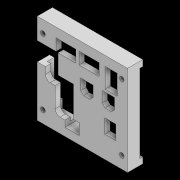
# Autodesk Inventor part: fan_controller_case_top
Saved by Autodesk Inventor 2022 (Build 260153000, 153)
## iProperties
Created: 2022-10-14
Part Number: fan_controller_case_top
Material: 一般
Document SubType Name: Modeling
Designer: numai
Density: 1 g/cm^3
Appearance: 既定
Author: numai
Autodesk Inventor part; units mm, degrees
ref_plane "YZ Plane" through (0, 0, 0) normal (1, 0, 0) x (0, 1, 0)
ref_plane "XZ Plane" through (0, 0, 0) normal (0, 1, 0) x (-1, 0, 0)
ref_plane "XY Plane" through (0, 0, 0) normal (0, 0, 1) x (1, 0, 0)
sketch "スケッチ1" plane through (0, 0, 0) normal (0, 0, 1) x (1, 0, 0)
  line L0 (-25.3, 21.7) -> (25.3, 21.7)
  line L1 (25.3, 21.7) -> (25.3, -21.7)
  line L2 (25.3, -21.7) -> (-25.3, -21.7)
  line L3 (-25.3, -21.7) -> (-25.3, 21.7)
  circle A0 centre (-22.1, 18.5) radius 1.3
  circle A1 centre (22.1, 18.5) radius 1.3
  circle A2 centre (22.1, -18.5) radius 1.3
  circle A3 centre (-22.1, -18.5) radius 1.3
  line L4 (-18.1, 19.2) -> (-18.1, 14.5)
  line L5 (-18.1, 14.5) -> (-22.8, 14.5)
  line L6 (-22.8, 14.5) -> (-22.8, -14.5)
  line L7 (-22.8, -14.5) -> (-18.1, -14.5)
  line L8 (-18.1, -14.5) -> (-18.1, -19.2)
  line L9 (-18.1, -19.2) -> (18.1, -19.2)
  line L10 (18.1, -19.2) -> (18.1, -14.5)
  line L11 (18.1, -14.5) -> (22.8, -14.5)
  line L12 (22.8, -14.5) -> (22.8, 14.5)
  line L13 (22.8, 14.5) -> (18.1, 14.5)
  line L14 (18.1, 14.5) -> (18.1, 19.2)
  line L15 (18.1, 19.2) -> (-18.1, 19.2)
  point P0 (0, 0)
  point P1 (0, 21.7)
  point P2 (-25.3, 0)
  dimension "d0" = 50.6
  dimension "d1" = 43.4
  dimension "d2" = 2.6
  dimension "d3" = 44.2
  dimension "d4" = 37
  dimension "d5" = 22.1
  dimension "d6" = 18.5
  dimension "d7" = 2.5
  dimension "d8" = 2.5
  dimension "d9" = 2.5
  dimension "d10" = 2.5
  dimension "d11" = 4
  dimension "d12" = 4
  dimension "d13" = 4
  dimension "d14" = 4
  dimension "d15" = 4
  constraints: 32 end point, 8 perpendicular, 6 point on line, 4 centre point, 3 equal radius, 3 horizontal alignment, 3 parallel, 3 vertical alignment, 2 midpoint, 1 horizontal, 1 vertical
  measures "d0" distance of L0.start L0.end
  measures "d1" distance of L0.end L1.end
  measures "d2" diameter of A0
  measures "d3" distance of A1.centre A0.centre
  measures "d4" distance of A3.centre A0.centre
  measures "d5" horizontal distance of point (0, 0) A1.centre
  measures "d6" vertical distance of point (0, 0) A0.centre
  measures "d7" distance between parallel lines of L0 L15
  measures "d8" distance between parallel lines of L3 L6
  measures "d9" distance between parallel lines of L2 L9
  measures "d10" distance between parallel lines of L1 L12
  measures "d11" distance from line of L5 A0.centre
  measures "d12" distance from line of L4 A0.centre
  measures "d13" distance from line of L14 A1.centre
  measures "d14" distance from line of A3.centre L7
  measures "d15" distance from line of L10 A2.centre
extrude "押し出し1" add sketch "スケッチ1" along normal blind 6.9
sketch "スケッチ4" plane through (0, 0, 6.9) normal (0, 0, 1) x (1, 0, 0)
  line L0 (-18.1, 14.5) -> (-18.1, 19.2) projected
  line L1 (-18.1, 19.2) -> (18.1, 19.2) projected
  line L2 (-22.8, 14.5) -> (-18.1, 14.5) projected
  line L3 (-22.8, -14.5) -> (-22.8, 14.5) projected
  line L4 (-18.1, -14.5) -> (-22.8, -14.5) projected
  line L5 (-18.1, -19.2) -> (-18.1, -14.5) projected
  line L6 (18.1, -19.2) -> (-18.1, -19.2) projected
  line L7 (18.1, -14.5) -> (18.1, -19.2) projected
  line L8 (22.8, -14.5) -> (18.1, -14.5) projected
  line L9 (22.8, 14.5) -> (22.8, -14.5) projected
  line L10 (18.1, 14.5) -> (22.8, 14.5) projected
  line L11 (18.1, 19.2) -> (18.1, 14.5) projected
  point P0 (0, 0)
extrude "押し出し4" add sketch "スケッチ4" against normal blind 3
sketch "スケッチ3" plane through (0, 0, 6.9) normal (0, 0, 1) x (1, 0, 0)
  line L0 (-14.6, 19.9) -> (-3.9, 19.9) construction
  line L1 (-3.9, 19.9) -> (-3.9, 13.6) construction
  line L2 (-3.9, 13.6) -> (-14.6, 13.6) construction
  line L3 (-14.6, 13.6) -> (-14.6, 19.9) construction
  line L4 (-1.6, 19.9) -> (9.1, 19.9) construction
  line L5 (9.1, 19.9) -> (9.1, 13.6) construction
  line L6 (9.1, 13.6) -> (-1.6, 13.6) construction
  line L7 (-1.6, 13.6) -> (-1.6, 19.9) construction
  line L8 (13, 19.8) -> (19.3, 19.8) construction
  line L9 (19.3, 19.8) -> (19.3, 9.1) construction
  line L10 (19.3, 9.1) -> (13, 9.1) construction
  line L11 (13, 9.1) -> (13, 19.8) construction
  line L12 (25.3, 21.7) -> (-25.3, 21.7) construction
  line L13 (25.3, -21.7) -> (25.3, 21.7) construction
  line L14 (-14.8, 13.4) -> (-3.7, 13.4)
  line L15 (-3.7, 13.4) -> (-3.7, 20.1)
  line L16 (-3.7, 20.1) -> (-14.8, 20.1)
  line L17 (-14.8, 20.1) -> (-14.8, 13.4)
  line L18 (-1.8, 13.4) -> (9.3, 13.4)
  line L19 (9.3, 13.4) -> (9.3, 20.1)
  line L20 (9.3, 20.1) -> (-1.8, 20.1)
  line L21 (-1.8, 20.1) -> (-1.8, 13.4)
  line L22 (12.8, 8.9) -> (19.5, 8.9)
  line L23 (19.5, 8.9) -> (19.5, 20)
  line L24 (19.5, 20) -> (12.8, 20)
  line L25 (12.8, 20) -> (12.8, 8.9)
  point P0 (0, 0)
  dimension "d20" = 6.3
  dimension "d21" = 10.7
  dimension "d23" = 6
  dimension "d24" = 1.8
  dimension "d25" = 26.9
  dimension "d26" = 39.9
  dimension "d27" = 12.6
  dimension "d28" = 0.2
  dimension "d29" = 0.2
  dimension "d30" = 0.2
  constraints: 48 end point, 12 parallel, 6 perpendicular, 3 equal length, 3 horizontal, 2 point on line, 9 other
  measures "d20" distance of L8.start L8.end
  measures "d21" distance of L8.end L9.end
  measures "d23" distance from line of L12.start L9
  measures "d24" distance between parallel lines of L12 L4
  measures "d25" distance between parallel lines of L13 L7
  measures "d26" distance from line of L12.start L3
  measures "d27" distance between parallel lines of L10 L12
  measures "d28" distance between parallel lines of L2 L14
  measures "d29" distance between parallel lines of L6 L18
  measures "d30" distance between parallel lines of L10 L22
extrude "押し出し3" cut sketch "スケッチ3" along normal through all both and the other way through all
sketch "スケッチ5" plane through (0, 0, 6.9) normal (0, 0, 1) x (1, 0, 0)
  line L0 (-21.5, 13.3) -> (-13.8, 13.3) construction
  line L1 (-13.8, 13.3) -> (-13.8, 3.3) construction
  line L2 (-13.8, 3.3) -> (-21.5, 3.3) construction
  line L3 (-21.5, 3.3) -> (-21.5, 13.3) construction
  line L4 (25.3, 21.7) -> (-25.3, 21.7) construction
  line L5 (25.3, -21.7) -> (25.3, 21.7) construction
  line L6 (-25.3, 13.5) -> (-13.6, 13.5)
  line L7 (-13.6, 13.5) -> (-13.6, 3.1)
  line L8 (-13.6, 3.1) -> (-25.3, 3.1)
  line L9 (-25.3, 3.1) -> (-25.3, 13.5)
  line L10 (-25.3, 21.7) -> (-25.3, -21.7) construction
  point P0 (0, 0)
  dimension "d35" = 46.8
  dimension "d36" = 7.7
  dimension "d37" = 18.4
  dimension "d38" = 10
  dimension "d39" = 0.2
  dimension "d40" = 0.2
  dimension "d41" = 0.2
  constraints: 16 end point, 4 parallel, 2 horizontal, 2 perpendicular, 1 point on line
  measures "d35" distance between parallel lines of L3 L5
  measures "d36" distance of L0.start L0.end
  measures "d37" distance between parallel lines of L2 L4
  measures "d38" distance of L2.end L0.start
  measures "d39" distance between parallel lines of L0 L6
  measures "d40" distance between parallel lines of L7 L1
  measures "d41" distance between parallel lines of L8 L2
extrude "押し出し5" cut sketch "スケッチ5" against normal through all
sketch "スケッチ6" plane through (0, 0, 6.9) normal (0, 0, 1) x (1, 0, 0)
  line L0 (-5.2, 2.3) -> (-15, 2.3) construction
  line L1 (-15, 2.3) -> (-15, -11.9) construction
  line L2 (-15, -11.9) -> (-5.2, -11.9) construction
  line L3 (-5.2, -11.9) -> (-5.2, 2.3) construction
  line L4 (25.3, 21.7) -> (-25.3, 21.7) construction
  line L5 (25.3, -21.7) -> (25.3, 21.7) construction
  line L6 (-15.2, 2.5) -> (-5, 2.5)
  line L7 (-5, 2.5) -> (-5, -12.1)
  line L8 (-5, -12.1) -> (-15.2, -12.1)
  line L9 (-15.2, -12.1) -> (-15.2, 2.5)
  point P0 (0, 0)
  dimension "d44" = 14.2
  dimension "d45" = 9.8
  dimension "d46" = 40.3
  dimension "d47" = 33.6
  dimension "d48" = 0.2
  constraints: 16 end point, 4 parallel, 2 perpendicular, 1 horizontal, 3 other
  measures "d44" distance of L2.end L0.start
  measures "d45" distance of L0.start L0.end
  measures "d46" distance between parallel lines of L5 L1
  measures "d47" distance between parallel lines of L2 L4
  measures "d48" distance between parallel lines of L0 L6
extrude "押し出し6" cut sketch "スケッチ6" against normal through all
sketch "スケッチ7" plane through (0, 0, 6.9) normal (0, 0, 1) x (1, 0, 0)
  line L0 (25.3, 21.7) -> (-25.3, 21.7) construction
  line L1 (25.3, -21.7) -> (25.3, 21.7) construction
  line L2 (12.8, -5.3) -> (18.6, -5.3) construction
  line L3 (18.6, -5.3) -> (18.6, -12.8) construction
  line L4 (18.6, -12.8) -> (12.8, -12.8) construction
  line L5 (12.8, -12.8) -> (12.8, -5.3) construction
  line L6 (-9.5, -14.8) -> (-2, -14.8) construction
  line L7 (-2, -14.8) -> (-2, -20.6) construction
  line L8 (-2, -20.6) -> (-9.5, -20.6) construction
  line L9 (-9.5, -20.6) -> (-9.5, -14.8) construction
  line L10 (12.6, -13) -> (18.8, -13)
  line L11 (18.8, -13) -> (18.8, -5.1)
  line L12 (18.8, -5.1) -> (12.6, -5.1)
  line L13 (12.6, -5.1) -> (12.6, -13)
  line L14 (-1.8, -20.8) -> (-1.8, -14.6)
  line L15 (-1.8, -14.6) -> (-9.7, -14.6)
  line L16 (-9.7, -14.6) -> (-9.7, -20.8)
  line L17 (-9.7, -20.8) -> (-1.8, -20.8)
  point P0 (0, 0)
  dimension "d51" = 7.5
  dimension "d52" = 5.8
  dimension "d53" = 12.5
  dimension "d54" = 34.5
  dimension "d55" = 42.3
  dimension "d56" = 34.8
  dimension "d57" = 0.2
  dimension "d58" = 0.2
  constraints: 32 end point, 8 parallel, 6 perpendicular, 2 horizontal, 6 other
  measures "d51" distance of L2.end L3.end
  measures "d52" distance of L2.start L2.end
  measures "d53" distance between parallel lines of L1 L5
  measures "d54" distance between parallel lines of L4 L0
  measures "d55" distance between parallel lines of L8 L0
  measures "d56" distance between parallel lines of L1 L9
  measures "d57" distance between parallel lines of L4 L10
  measures "d58" distance between parallel lines of L7 L14
extrude "押し出し7" cut sketch "スケッチ7" against normal through all
sketch "スケッチ8" plane through (0, 0, 6.9) normal (0, 0, 1) x (1, 0, 0)
  circle A0 centre (-18, -0.6) radius 2.5 construction
  circle A1 centre (-12.5, -14.6) radius 2.5 construction
  line L0 (25.3, 21.7) -> (-25.3, 21.7) construction
  line L1 (25.3, -21.7) -> (25.3, 21.7) construction
  circle A2 centre (-18, -0.6) radius 2.7
  circle A3 centre (-12.5, -14.6) radius 2.7
  point P0 (0, 0)
  dimension "d61" = 5
  dimension "d62" = 22.3
  dimension "d63" = 36.3
  dimension "d64" = 43.3
  dimension "d65" = 37.8
  dimension "d66" = 0.2
  dimension "d67" = 0.2
  constraints: 4 centre point, 1 equal radius
  measures "d61" diameter of A0
  measures "d62" distance from line of A0.centre L0
  measures "d63" distance from line of A1.centre L0
  measures "d64" distance from line of L1 A0.centre
  measures "d65" distance from line of L1 A1.centre
  measures "d66" radial gap between concentric circles of A0 A2
  measures "d67" radial gap between concentric circles of A1 A3
extrude "押し出し8" cut sketch "スケッチ8" against normal through all
sketch "スケッチ9" plane through (0, 0, 6.9) normal (0, 0, 1) x (1, 0, 0)
  line L0 (11.3, 1.5) -> (11.3, 7.3) construction
  line L1 (11.3, 7.3) -> (17.8, 7.3) construction
  line L2 (17.8, 7.3) -> (17.8, 1.5) construction
  line L3 (17.8, 1.5) -> (16.3, 0) construction
  line L4 (16.3, 0) -> (12.8, 0) construction
  line L5 (12.8, 0) -> (11.3, 1.5) construction
  line L6 (-0.7, 1.5) -> (-0.7, 7.3) construction
  line L7 (-0.7, 7.3) -> (5.8, 7.3) construction
  line L8 (5.8, 7.3) -> (5.8, 1.5) construction
  line L9 (5.8, 1.5) -> (4.3, 0) construction
  line L10 (4.3, 0) -> (0.8, 0) construction
  line L11 (0.8, 0) -> (-0.7, 1.5) construction
  line L12 (25.3, -21.7) -> (25.3, 21.7) construction
  line L13 (25.3, 21.7) -> (-25.3, 21.7) construction
  line L14 (6, 7.5) -> (-0.9, 7.5)
  line L15 (-0.9, 7.5) -> (-0.9, 1.4172)
  line L16 (-0.9, 1.4172) -> (0.7172, -0.2)
  line L17 (0.7172, -0.2) -> (4.3828, -0.2)
  line L18 (4.3828, -0.2) -> (6, 1.4172)
  line L19 (6, 1.4172) -> (6, 7.5)
  line L20 (18, 7.5) -> (11.1, 7.5)
  line L21 (11.1, 7.5) -> (11.1, 1.4172)
  line L22 (11.1, 1.4172) -> (12.7172, -0.2)
  line L23 (12.7172, -0.2) -> (16.3828, -0.2)
  line L24 (16.3828, -0.2) -> (18, 1.4172)
  line L25 (18, 1.4172) -> (18, 7.5)
  point P0 (0, 0)
  dimension "d70" = 135
  dimension "d71" = 135
  dimension "d72" = 135
  dimension "d73" = 135
  dimension "d74" = 7.3
  dimension "d75" = 6.5
  dimension "d76" = 1.5
  dimension "d77" = 26
  dimension "d78" = 14
  dimension "d79" = 21.7
  dimension "d80" = 0.2
  dimension "d81" = 0.2
  constraints: 48 end point, 8 perpendicular, 5 equal length, 4 parallel, 2 vertical, 1 horizontal alignment, 10 other
  measures "d70" angle of L2 L3
  measures "d71" angle of L5 L0
  measures "d72" angle of L8 L9
  measures "d73" angle of L11 L6
  measures "d74" distance between parallel lines of L10 L7
  measures "d75" distance between parallel lines of L8 L6
  measures "d76" horizontal distance of L9.end L8.end
  measures "d77" distance between parallel lines of L12 L6
  measures "d78" distance between parallel lines of L12 L0
  measures "d79" distance between parallel lines of L4 L13
  measures "d80" distance between parallel lines of L7 L14
  measures "d81" distance between parallel lines of L1 L20
extrude "押し出し9" cut sketch "スケッチ9" against normal through all
sketch "スケッチ10" plane through (0, 0, 6.9) normal (0, 0, 1) x (1, 0, 0)
  arc A0 (-13.5198, -12.1) -> (-11.4802, -12.1) centre (-12.5, -14.6) ccw construction
  circle A1 centre (-18, -0.6) radius 2.7 construction
  line L0 (-13.6, 13.4) -> (-13.6, 3.1) construction
  line L1 (-15.2, -12.1) -> (-15.2, 2.5) construction
  line L2 (-9.7, -14.6) -> (-1.8, -14.6) construction
  line L3 (-12.5, -14.6) -> (-15.2, -14.6) construction
  line L4 (-5, -14.6881) -> (-5, -8.3419)
  line L5 (-5, -8.3419) -> (-15.2, -8.3419)
  line L6 (-15.2, -8.3419) -> (-15.2, -14.6)
  line L7 (-15.2, -14.6) -> (-12.5, -14.6)
  line L8 (-12.5, -14.6) -> (-12.5, -17.3)
  line L9 (-12.5, -17.3) -> (-5, -17.3)
  line L10 (-5, -17.3) -> (-5, -14.6881)
  line L11 (-9.7, -20.8) -> (-9.7, -14.6) construction
  line L12 (-20.7, 3.1) -> (-20.7, -0.6)
  line L13 (-20.7, -0.6) -> (-18, -0.6)
  line L14 (-18, -0.6) -> (-18, -3.3)
  line L15 (-18, -3.3) -> (-13.6, -3.3)
  line L16 (-13.6, -3.3) -> (-13.6, 3.1)
  line L17 (-13.6, 3.1) -> (-20.7, 3.1)
  point P0 (0, 0)
  point P1 (-5, -12.1)
  constraints: 28 end point, 6 perpendicular, 4 point on circle, 3 horizontal, 2 collinear, 1 coincident, 1 parallel, 1 point on line, 1 vertical
extrude "押し出し10" cut sketch "スケッチ10" against normal through all
sketch "スケッチ11" plane through (-25.3, 21.7, 0) normal (0, 1, 0) x (1, 0, 0)
  line L0 (50.6, -6.9) -> (0, -6.9) projected
  line L1 (50.6, 0) -> (50.6, -6.9) projected
  line L2 (50.6, 0) -> (0, 0) projected
  line L3 (0, 0) -> (0, -6.9) projected
  point P0 (25.3, 0)
extrude "押し出し11" add sketch "スケッチ11" along normal blind 3.6
sketch "スケッチ12" plane through (-25.3, -21.7, 0) normal (0, -1, 0) x (1, 0, 0)
  line L0 (0, 0) -> (0, 6.9) projected
  line L1 (0, 0) -> (50.6, 0) projected
  line L2 (0, 6.9) -> (50.6, 6.9) projected
  line L3 (50.6, 0) -> (50.6, 6.9) projected
  point P0 (25.3, 0)
extrude "押し出し12" add sketch "スケッチ12" along normal blind 3.6
sketch "スケッチ13" plane through (0, 0, 0) normal (0, 0, -1) x (-1, 0, 0)
  line L0 (-25.3, 25.3) -> (25.3, 25.3) projected
  line L1 (25.3, -25.3) -> (-25.3, -25.3) projected
  line L2 (-25.3, 21.9) -> (25.3, 21.9)
  line L3 (25.3, -21.9) -> (-25.3, -21.9)
  line L4 (25.3, 21.9) -> (25.3, 25.3)
  line L5 (-25.3, 25.3) -> (-25.3, 21.9)
  line L6 (25.3, -21.9) -> (25.3, -25.3)
  line L7 (-25.3, -21.9) -> (-25.3, -25.3)
  point P0 (0, 0)
  dimension "d90" = 3.4
  dimension "d91" = 3.4
  constraints: 12 end point, 3 vertical, 2 parallel, 1 perpendicular
  measures "d90" distance between parallel lines of L0 L2
  measures "d91" distance between parallel lines of L1 L3
extrude "押し出し13" add sketch "スケッチ13" along normal blind 1.6
equation "\"d5\" = 0.5 * d3"
equation "\"d6\" = 0.5 * d4"
equation "\"d8\" = d7"
equation "\"d9\" = d7"
equation "\"d10\" = d7"
equation "\"d12\" = d11"
equation "\"d13\" = d11"
equation "\"d14\" = d11"
equation "\"d15\" = d11"
equation "\"d40\" = d39"
equation "\"d41\" = d39"
equation "\"d71\" = d70"
equation "\"d73\" = d72"
equation "\"d81\" = d80"
